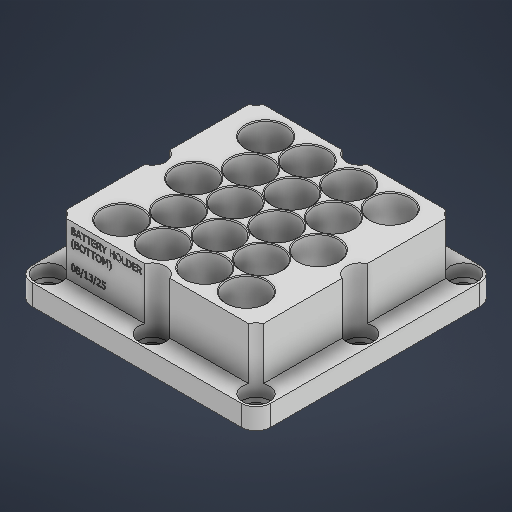
# Autodesk Inventor part: Battery Holder
Saved by Autodesk Inventor 2025 (Build 290162000, 162)
## iProperties
Created: 2025-08-08
Part Number: Battery Holder
Material: Generic
Document SubType Name: Modeling
Designer: mayhe
Density: 1 g/cm^3
Appearance: Default
Author: mayhe
Autodesk Inventor part; units mm, degrees
ref_plane "YZ Plane" through (0, 0, 0) normal (1, 0, 0) x (0, 1, 0)
ref_plane "XZ Plane" through (0, 0, 0) normal (0, 1, 0) x (-1, 0, 0)
ref_plane "XY Plane" through (0, 0, 0) normal (0, 0, 1) x (1, 0, 0)
sketch "Sketch1" plane through (0, 0, 0) normal (0, 1, 0) x (-1, 0, 0)
  line L0 (57.5, 57.5) -> (-57.5, 57.5)
  line L1 (-57.5, 57.5) -> (-57.5, -57.5)
  line L2 (-57.5, -57.5) -> (57.5, -57.5)
  line L3 (57.5, -57.5) -> (57.5, 57.5)
  line L4 (57.5, 57.5) -> (-57.5, -57.5) construction
  line L5 (-57.5, 57.5) -> (57.5, -57.5) construction
  point P0 (0, 0)
  dimension "d0" = 115
  dimension "d1" = 115
  constraints: 12 end point, 2 midpoint, 2 parallel, 1 horizontal, 1 perpendicular
  measures "d0" distance of L2.end L1.end
  measures "d1" distance of L1.end L0.end
extrude "Extrusion1" add sketch "Sketch1" along normal blind 10
sketch "Sketch4" plane through (0, 10, 0) normal (0, 1, 0) x (1, 0, 0)
  line L0 (-47.5, -47.5) -> (47.5, -47.5)
  line L1 (47.5, -47.5) -> (47.5, 47.5)
  line L2 (47.5, 47.5) -> (-47.5, 47.5)
  line L3 (-47.5, 47.5) -> (-47.5, -47.5)
  line L4 (-57.5, 57.5) -> (-57.5, -57.5) projected
  line L5 (-57.5, 0) -> (-47.5, 0)
  line L6 (-30, 34.641) -> (30, 34.641)
  line L7 (30, 34.641) -> (30, -34.641)
  line L8 (30, -34.641) -> (-30, -34.641)
  line L9 (-30, -34.641) -> (-30, 34.641)
  line L10 (-30, 34.641) -> (30, -34.641) construction
  line L11 (30, 34.641) -> (-30, -34.641) construction
  circle A0 centre (-30, 34.641) radius 9.5
  circle A1 centre (-10, 34.641) radius 9.5
  circle A2 centre (10, 34.641) radius 9.5
  circle A3 centre (30, 34.641) radius 9.5
  circle A4 centre (-30, 0) radius 9.5
  circle A5 centre (-10, 0) radius 9.5
  circle A6 centre (10, 0) radius 9.5
  circle A7 centre (30, 0) radius 9.5
  circle A8 centre (-30, -34.641) radius 9.5
  circle A9 centre (-10, -34.641) radius 9.5
  circle A10 centre (10, -34.641) radius 9.5
  circle A11 centre (30, -34.641) radius 9.5
  circle A12 centre (-20, 17.3205) radius 9.5
  circle A13 centre (0, 17.3205) radius 9.5
  circle A14 centre (20, 17.3205) radius 9.5
  circle A15 centre (-20, -17.3205) radius 9.5
  circle A16 centre (0, -17.3205) radius 9.5
  circle A17 centre (20, -17.3205) radius 9.5
  point P0 (47.3285, -94.6135)
  point P1 (-53.5957, 219.1108)
  point P2 (0, 0)
  dimension "d1" = 115
  dimension "d138" = 3
  dimension "d48" = 95
  dimension "d49" = 95
  dimension "d132" = 60
  dimension "d133" = 69.282
  dimension "d134" = 19
  dimension "d137" = 20
  dimension "d140" = 34.641
  dimension "d143" = 19
  dimension "d146" = 10
  dimension "d147" = 17.3205
  dimension "d150" = 20
  dimension "d153" = 34.641
  constraints: 22 end point, 18 centre point, 4 horizontal, 4 midpoint, 4 parallel, 2 perpendicular, 2 vertical, 1 coincident, 32 other
  measures "d48" distance of L2.end L1.end
  measures "d49" distance of L1.end L0.end
  measures "d132" distance of L7.end L8.end
  measures "d133" distance of L6.end L7.end
  measures "d134" diameter of A0
  measures "d137" distance of A0.centre A1.centre
  measures "d140" distance of A0.centre A4.centre
  measures "d143" diameter of A12
  measures "d146" horizontal distance of A1.centre A12.centre
  measures "d147" vertical distance of A12.centre A1.centre
  measures "d150" distance of A12.centre A13.centre
  measures "d153" distance of A12.centre A15.centre
extrude "Extrusion2" add sketch "Sketch4" along normal blind 25 contours L3 L2 L1 L0 | L6 A1 A2 A3 L7 A7 A11 L8 A10 A9 A8 L9 A4 A0
sketch "Sketch5" plane through (0, 35, 0) normal (0, 1, 0) x (1, 0, 0)
  line L0 (50, 50) -> (-50, 50)
  line L1 (-50, 50) -> (-50, -50)
  line L2 (-50, -50) -> (50, -50)
  line L3 (50, -50) -> (50, 50)
  line L4 (50, 50) -> (-50, -50) construction
  line L5 (-50, 50) -> (50, -50) construction
  circle A0 centre (-50, -50) radius 3.5
  circle A1 centre (0, -50) radius 3.5
  circle A2 centre (-50, 0) radius 3.5
  circle A3 centre (0, 0) radius 3.5
  circle A4 centre (50, -50) radius 3.5
  circle A5 centre (50, 0) radius 3.5
  circle A6 centre (-50, 50) radius 3.5
  circle A7 centre (0, 50) radius 3.5
  circle A8 centre (50, 50) radius 3.5
  point P0 (0, 0)
  dimension "d156" = 100
  dimension "d157" = 100
  dimension "d158" = 7
  dimension "d161" = 50
  dimension "d164" = 50
  constraints: 12 end point, 9 centre point, 2 horizontal, 2 midpoint, 2 parallel, 1 coincident, 1 perpendicular, 1 vertical, 16 other
  measures "d156" distance of L2.end L1.end
  measures "d157" distance of L1.end L0.end
  measures "d158" diameter of A0
  measures "d161" distance of A0.centre A1.centre
  measures "d164" distance of A0.centre A2.centre
hole "Hole3" at (-50, 35, 50) at (50, 35, 50) at (-50, 35, -50) at (50, 35, -50) at (-50, 35, 0) at (0, 35, 50) at (50, 35, 0) at (0, 35, -50) direction (0, -1, 0) diameter 7.125 end through all counterbore diameter 13 counterbore depth 31
fillet "Fillet1" radius 7.125 4 edges at (57.5, 5, 57.5) (57.5, 5, -57.5) (-57.5, 5, 57.5) (-57.5, 5, -57.5)
chamfer "Chamfer1" distance 0.4 angle 45 18 edges at (-39.5, 35, -34.641) (-19.5, 35, -34.641) (-29.5, 35, -17.3205) (0.5, 35, -34.641) (20.5, 35, -34.641) (10.5, 35, -17.3205) (-9.5, 35, -17.3205) (-39.5, 35, 0) (-19.5, 35, 0) (0.5, 35, 0) (20.5, 35, 0) (10.5, 35, 17.3205) (-9.5, 35, 17.3205) (-29.5, 35, 17.3205) (-39.5, 35, 34.641) (-19.5, 35, 34.641) (0.5, 35, 34.641) (20.5, 35, 34.641)
sketch "Sketch6" plane through (-44, 10, 47.5) normal (0, 0, 1) x (1, 0, 0)
  line L0 (2.3115, 22.6775) -> (39.9401, 22.6775) construction
  line L1 (39.9401, 22.6775) -> (39.9401, -1.6821) construction
  line L2 (39.9401, -1.6821) -> (2.3115, -1.6821) construction
  line L3 (2.3115, -1.6821) -> (2.3115, 22.6775) construction
  spline S0 degree 2 poles (4.6876, 20.5014) (4.6876, 20.2741) (4.5147, 19.9259) (4.3715, 19.8123) knots 0 0 0 1 2 2 2
  spline S1 degree 2 poles (4.3715, 19.8123) (4.1986, 19.6789) (3.8058, 19.5653) (3.4946, 19.5653) knots 0 0 0 1 2 2 2
  line L4 (3.4946, 19.5653) -> (2.6202, 19.5653)
  line L5 (2.6202, 19.5653) -> (2.6202, 22.6133)
  line L6 (2.6202, 22.6133) -> (3.4279, 22.6133)
  spline S2 degree 2 poles (3.4279, 22.6133) (3.754, 22.6133) (4.08, 22.5713) (4.2282, 22.4898) knots 0 0 0 1 2 2 2
  spline S3 degree 2 poles (4.2282, 22.4898) (4.3937, 22.4033) (4.5444, 22.1193) (4.5444, 21.9266) knots 0 0 0 1 2 2 2
  spline S4 degree 2 poles (4.5444, 21.9266) (4.5444, 21.7117) (4.3171, 21.3708) (4.117, 21.2745) knots 0 0 0 1 2 2 2
  line L7 (4.117, 21.2745) -> (4.117, 21.2597)
  spline S5 degree 2 poles (4.117, 21.2597) (4.3887, 21.1856) (4.6876, 20.7929) (4.6876, 20.5014) knots 0 0 0 1 2 2 2
  spline S6 degree 2 poles (4.2652, 20.4841) (4.2652, 20.657) (4.1664, 20.8793) (4.0182, 20.9583) knots 0 0 0 1 2 2 2
  spline S7 degree 2 poles (4.0182, 20.9583) (3.9219, 21.0077) (3.6947, 21.0374) (3.4847, 21.0374) knots 0 0 0 1 2 2 2
  line L8 (3.4847, 21.0374) -> (3.0253, 21.0374)
  line L9 (3.0253, 21.0374) -> (3.0253, 19.9111)
  line L10 (3.0253, 19.9111) -> (3.3538, 19.9111)
  spline S8 degree 2 poles (3.3538, 19.9111) (3.6206, 19.9111) (3.9269, 19.9605) (4.0454, 20.0395) knots 0 0 0 1 2 2 2
  spline S9 degree 2 poles (4.0454, 20.0395) (4.159, 20.121) (4.2652, 20.3235) (4.2652, 20.4841) knots 0 0 0 1 2 2 2
  spline S10 degree 2 poles (4.122, 21.8698) (4.122, 21.9785) (4.0479, 22.1415) (3.9664, 22.1884) knots 0 0 0 1 2 2 2
  spline S11 degree 2 poles (3.9664, 22.1884) (3.8676, 22.2428) (3.628, 22.2675) (3.4131, 22.2675) knots 0 0 0 1 2 2 2
  line L11 (3.4131, 22.2675) -> (3.0253, 22.2675)
  line L12 (3.0253, 22.2675) -> (3.0253, 21.3758)
  line L13 (3.0253, 21.3758) -> (3.4847, 21.3758)
  spline S12 degree 2 poles (3.4847, 21.3758) (3.6749, 21.3758) (3.8552, 21.4153) (3.9516, 21.477) knots 0 0 0 1 2 2 2
  spline S13 degree 2 poles (3.9516, 21.477) (4.0454, 21.5363) (4.122, 21.7265) (4.122, 21.8698) knots 0 0 0 1 2 2 2
  line L14 (4.7617, 19.5653) -> (5.7892, 22.6133)
  line L15 (5.7892, 22.6133) -> (6.2882, 22.6133)
  line L16 (6.2882, 22.6133) -> (7.3157, 19.5653)
  line L17 (7.3157, 19.5653) -> (6.8884, 19.5653)
  line L18 (6.8884, 19.5653) -> (6.6118, 20.4174)
  line L19 (6.6118, 20.4174) -> (5.4484, 20.4174)
  line L20 (5.4484, 20.4174) -> (5.1717, 19.5653)
  line L21 (5.1717, 19.5653) -> (4.7617, 19.5653)
  line L22 (6.5006, 20.7632) -> (6.0288, 22.1983)
  line L23 (6.0288, 22.1983) -> (5.5595, 20.7632)
  line L24 (5.5595, 20.7632) -> (6.5006, 20.7632)
  line L25 (8.3161, 19.5653) -> (8.3161, 22.2526)
  line L26 (8.3161, 22.2526) -> (7.2935, 22.2526)
  line L27 (7.2935, 22.2526) -> (7.2935, 22.6133)
  line L28 (7.2935, 22.6133) -> (9.7437, 22.6133)
  line L29 (9.7437, 22.6133) -> (9.7437, 22.2526)
  line L30 (9.7437, 22.2526) -> (8.7212, 22.2526)
  line L31 (8.7212, 22.2526) -> (8.7212, 19.5653)
  line L32 (8.7212, 19.5653) -> (8.3161, 19.5653)
  line L33 (10.7639, 19.5653) -> (10.7639, 22.2526)
  line L34 (10.7639, 22.2526) -> (9.7413, 22.2526)
  line L35 (9.7413, 22.2526) -> (9.7413, 22.6133)
  line L36 (9.7413, 22.6133) -> (12.1915, 22.6133)
  line L37 (12.1915, 22.6133) -> (12.1915, 22.2526)
  line L38 (12.1915, 22.2526) -> (11.1689, 22.2526)
  line L39 (11.1689, 22.2526) -> (11.1689, 19.5653)
  line L40 (11.1689, 19.5653) -> (10.7639, 19.5653)
  line L41 (12.5003, 19.5653) -> (12.5003, 22.6133)
  line L42 (12.5003, 22.6133) -> (14.4071, 22.6133)
  line L43 (14.4071, 22.6133) -> (14.4071, 22.2526)
  line L44 (14.4071, 22.2526) -> (12.9054, 22.2526)
  line L45 (12.9054, 22.2526) -> (12.9054, 21.4178)
  line L46 (12.9054, 21.4178) -> (14.3059, 21.4178)
  line L47 (14.3059, 21.4178) -> (14.3059, 21.0571)
  line L48 (14.3059, 21.0571) -> (12.9054, 21.0571)
  line L49 (12.9054, 21.0571) -> (12.9054, 19.9259)
  line L50 (12.9054, 19.9259) -> (14.4071, 19.9259)
  line L51 (14.4071, 19.9259) -> (14.4071, 19.5653)
  line L52 (14.4071, 19.5653) -> (12.5003, 19.5653)
  line L53 (17.2106, 19.5653) -> (16.6845, 19.5653)
  line L54 (16.6845, 19.5653) -> (15.7212, 20.778)
  line L55 (15.7212, 20.778) -> (15.2568, 20.778)
  line L56 (15.2568, 20.778) -> (15.2568, 19.5653)
  line L57 (15.2568, 19.5653) -> (14.8517, 19.5653)
  line L58 (14.8517, 19.5653) -> (14.8517, 22.6133)
  line L59 (14.8517, 22.6133) -> (15.6372, 22.6133)
  spline S14 degree 2 poles (15.6372, 22.6133) (15.899, 22.6133) (16.2522, 22.5564) (16.4128, 22.4527) knots 0 0 0 1 2 2 2
  spline S15 degree 2 poles (16.4128, 22.4527) (16.5733, 22.349) (16.7586, 22.0254) (16.7586, 21.7858) knots 0 0 0 1 2 2 2
  spline S16 degree 2 poles (16.7586, 21.7858) (16.7586, 21.4523) (16.4177, 21.0003) (16.1263, 20.8917) knots 0 0 0 1 2 2 2
  line L60 (16.1263, 20.8917) -> (17.2106, 19.5653)
  spline S17 degree 2 poles (16.3362, 21.7537) (16.3362, 21.8871) (16.2424, 22.0921) (16.1436, 22.1588) knots 0 0 0 1 2 2 2
  spline S18 degree 2 poles (16.1436, 22.1588) (16.0571, 22.2156) (15.8274, 22.2625) (15.6594, 22.2625) knots 0 0 0 1 2 2 2
  line L61 (15.6594, 22.2625) -> (15.2568, 22.2625)
  line L62 (15.2568, 22.2625) -> (15.2568, 21.1164)
  line L63 (15.2568, 21.1164) -> (15.6125, 21.1164)
  spline S19 degree 2 poles (15.6125, 21.1164) (15.7879, 21.1164) (16.067, 21.1782) (16.1633, 21.2745) knots 0 0 0 1 2 2 2
  spline S20 degree 2 poles (16.1633, 21.2745) (16.2522, 21.3585) (16.3362, 21.5956) (16.3362, 21.7537) knots 0 0 0 1 2 2 2
  line L64 (19.5868, 22.6133) -> (18.5568, 20.9139)
  line L65 (18.5568, 20.9139) -> (18.5568, 19.5653)
  line L66 (18.5568, 19.5653) -> (18.1517, 19.5653)
  line L67 (18.1517, 19.5653) -> (18.1517, 20.8719)
  line L68 (18.1517, 20.8719) -> (17.1217, 22.6133)
  line L69 (17.1217, 22.6133) -> (17.5712, 22.6133)
  line L70 (17.5712, 22.6133) -> (18.3592, 21.272)
  line L71 (18.3592, 21.272) -> (19.157, 22.6133)
  line L72 (19.157, 22.6133) -> (19.5868, 22.6133)
  line L73 (23.3906, 19.5653) -> (22.9855, 19.5653)
  line L74 (22.9855, 19.5653) -> (22.9855, 21.0571)
  line L75 (22.9855, 21.0571) -> (21.5825, 21.0571)
  line L76 (21.5825, 21.0571) -> (21.5825, 19.5653)
  line L77 (21.5825, 19.5653) -> (21.1774, 19.5653)
  line L78 (21.1774, 19.5653) -> (21.1774, 22.6133)
  line L79 (21.1774, 22.6133) -> (21.5825, 22.6133)
  line L80 (21.5825, 22.6133) -> (21.5825, 21.4178)
  line L81 (21.5825, 21.4178) -> (22.9855, 21.4178)
  line L82 (22.9855, 21.4178) -> (22.9855, 22.6133)
  line L83 (22.9855, 22.6133) -> (23.3906, 22.6133)
  line L84 (23.3906, 22.6133) -> (23.3906, 19.5653)
  spline S21 degree 2 poles (26.1644, 22.265) (26.3373, 22.0624) (26.53, 21.4696) (26.53, 21.0893) knots 0 0 0 1 2 2 2
  spline S22 degree 2 poles (26.53, 21.0893) (26.53, 20.7188) (26.3423, 20.1185) (26.1644, 19.916) knots 0 0 0 1 2 2 2
  spline S23 degree 2 poles (26.1644, 19.916) (25.9767, 19.7036) (25.4802, 19.501) (25.1813, 19.501) knots 0 0 0 1 2 2 2
  spline S24 degree 2 poles (25.1813, 19.501) (24.8726, 19.501) (24.3786, 19.711) (24.1983, 19.916) knots 0 0 0 1 2 2 2
  spline S25 degree 2 poles (24.1983, 19.916) (24.0229, 20.1185) (23.8352, 20.7138) (23.8352, 21.0893) knots 0 0 0 1 2 2 2
  spline S26 degree 2 poles (23.8352, 21.0893) (23.8352, 21.4721) (24.0254, 22.055) (24.2007, 22.265) knots 0 0 0 1 2 2 2
  spline S27 degree 2 poles (24.2007, 22.265) (24.3786, 22.4675) (24.8751, 22.6775) (25.1813, 22.6775) knots 0 0 0 1 2 2 2
  spline S28 degree 2 poles (25.1813, 22.6775) (25.4926, 22.6775) (25.9915, 22.4601) (26.1644, 22.265) knots 0 0 0 1 2 2 2
  spline S29 degree 2 poles (26.1076, 21.0893) (26.1076, 21.3906) (25.9767, 21.8574) (25.8581, 22.0106) knots 0 0 0 1 2 2 2
  spline S30 degree 2 poles (25.8581, 22.0106) (25.7371, 22.1687) (25.3962, 22.3267) (25.1838, 22.3267) knots 0 0 0 1 2 2 2
  spline S31 degree 2 poles (25.1838, 22.3267) (24.964, 22.3267) (24.633, 22.1736) (24.507, 22.0106) knots 0 0 0 1 2 2 2
  spline S32 degree 2 poles (24.507, 22.0106) (24.386, 21.855) (24.2576, 21.3857) (24.2576, 21.0893) knots 0 0 0 1 2 2 2
  spline S33 degree 2 poles (24.2576, 21.0893) (24.2576, 20.489) (24.7614, 19.8518) (25.1838, 19.8518) knots 0 0 0 1 2 2 2
  spline S34 degree 2 poles (25.1838, 19.8518) (25.6062, 19.8518) (26.1076, 20.489) (26.1076, 21.0893) knots 0 0 0 1 2 2 2
  line L85 (28.7406, 19.5653) -> (26.9746, 19.5653)
  line L86 (26.9746, 19.5653) -> (26.9746, 22.6133)
  line L87 (26.9746, 22.6133) -> (27.3797, 22.6133)
  line L88 (27.3797, 22.6133) -> (27.3797, 19.9259)
  line L89 (27.3797, 19.9259) -> (28.7406, 19.9259)
  line L90 (28.7406, 19.9259) -> (28.7406, 19.5653)
  spline S35 degree 2 poles (31.4626, 21.0868) (31.4626, 20.6694) (31.1242, 19.9975) (30.8402, 19.8098) knots 0 0 0 1 2 2 2
  spline S36 degree 2 poles (30.8402, 19.8098) (30.608, 19.6641) (30.1313, 19.5653) (29.7608, 19.5653) knots 0 0 0 1 2 2 2
  line L91 (29.7608, 19.5653) -> (29.0593, 19.5653)
  line L92 (29.0593, 19.5653) -> (29.0593, 22.6133)
  line L93 (29.0593, 22.6133) -> (29.7533, 22.6133)
  spline S37 degree 2 poles (29.7533, 22.6133) (30.1831, 22.6133) (30.6722, 22.4848) (30.8451, 22.3712) knots 0 0 0 1 2 2 2
  spline S38 degree 2 poles (30.8451, 22.3712) (31.139, 22.1761) (31.4626, 21.5314) (31.4626, 21.0868) knots 0 0 0 1 2 2 2
  spline S39 degree 2 poles (31.0402, 21.0917) (31.0402, 21.4425) (30.808, 21.9389) (30.5783, 22.0797) knots 0 0 0 1 2 2 2
  spline S40 degree 2 poles (30.5783, 22.0797) (30.4153, 22.1761) (30.0473, 22.2625) (29.7731, 22.2625) knots 0 0 0 1 2 2 2
  line L94 (29.7731, 22.2625) -> (29.4644, 22.2625)
  line L95 (29.4644, 22.2625) -> (29.4644, 19.916)
  line L96 (29.4644, 19.916) -> (29.7731, 19.916)
  spline S41 degree 2 poles (29.7731, 19.916) (30.0423, 19.916) (30.4499, 20.0024) (30.6154, 20.1185) knots 0 0 0 1 2 2 2
  spline S42 degree 2 poles (30.6154, 20.1185) (30.8278, 20.2618) (31.0402, 20.736) (31.0402, 21.0917) knots 0 0 0 1 2 2 2
  line L97 (31.9023, 19.5653) -> (31.9023, 22.6133)
  line L98 (31.9023, 22.6133) -> (33.8091, 22.6133)
  line L99 (33.8091, 22.6133) -> (33.8091, 22.2526)
  line L100 (33.8091, 22.2526) -> (32.3073, 22.2526)
  line L101 (32.3073, 22.2526) -> (32.3073, 21.4178)
  line L102 (32.3073, 21.4178) -> (33.7078, 21.4178)
  line L103 (33.7078, 21.4178) -> (33.7078, 21.0571)
  line L104 (33.7078, 21.0571) -> (32.3073, 21.0571)
  line L105 (32.3073, 21.0571) -> (32.3073, 19.9259)
  line L106 (32.3073, 19.9259) -> (33.8091, 19.9259)
  line L107 (33.8091, 19.9259) -> (33.8091, 19.5653)
  line L108 (33.8091, 19.5653) -> (31.9023, 19.5653)
  line L109 (36.6126, 19.5653) -> (36.0865, 19.5653)
  line L110 (36.0865, 19.5653) -> (35.1232, 20.778)
  line L111 (35.1232, 20.778) -> (34.6588, 20.778)
  line L112 (34.6588, 20.778) -> (34.6588, 19.5653)
  line L113 (34.6588, 19.5653) -> (34.2537, 19.5653)
  line L114 (34.2537, 19.5653) -> (34.2537, 22.6133)
  line L115 (34.2537, 22.6133) -> (35.0392, 22.6133)
  spline S43 degree 2 poles (35.0392, 22.6133) (35.301, 22.6133) (35.6542, 22.5564) (35.8148, 22.4527) knots 0 0 0 1 2 2 2
  spline S44 degree 2 poles (35.8148, 22.4527) (35.9753, 22.349) (36.1606, 22.0254) (36.1606, 21.7858) knots 0 0 0 1 2 2 2
  spline S45 degree 2 poles (36.1606, 21.7858) (36.1606, 21.4523) (35.8197, 21.0003) (35.5282, 20.8917) knots 0 0 0 1 2 2 2
  line L116 (35.5282, 20.8917) -> (36.6126, 19.5653)
  spline S46 degree 2 poles (35.7382, 21.7537) (35.7382, 21.8871) (35.6443, 22.0921) (35.5455, 22.1588) knots 0 0 0 1 2 2 2
  spline S47 degree 2 poles (35.5455, 22.1588) (35.4591, 22.2156) (35.2294, 22.2625) (35.0614, 22.2625) knots 0 0 0 1 2 2 2
  line L117 (35.0614, 22.2625) -> (34.6588, 22.2625)
  line L118 (34.6588, 22.2625) -> (34.6588, 21.1164)
  line L119 (34.6588, 21.1164) -> (35.0145, 21.1164)
  spline S48 degree 2 poles (35.0145, 21.1164) (35.1899, 21.1164) (35.469, 21.1782) (35.5653, 21.2745) knots 0 0 0 1 2 2 2
  spline S49 degree 2 poles (35.5653, 21.2745) (35.6542, 21.3585) (35.7382, 21.5956) (35.7382, 21.7537) knots 0 0 0 1 2 2 2
  line L120 (3.7638, 13.7045) -> (3.2945, 13.7045)
  spline S50 degree 2 poles (3.2945, 13.7045) (2.9389, 14.1269) (2.5313, 15.0729) (2.5313, 15.7176) knots 0 0 0 1 2 2 2
  spline S51 degree 2 poles (2.5313, 15.7176) (2.5313, 16.3474) (2.9339, 17.3083) (3.2945, 17.7307) knots 0 0 0 1 2 2 2
  line L121 (3.2945, 17.7307) -> (3.7638, 17.7307)
  line L122 (3.7638, 17.7307) -> (3.7638, 17.7109)
  spline S52 degree 2 poles (3.7638, 17.7109) (3.5983, 17.5602) (3.297, 17.17) (3.1686, 16.9106) knots 0 0 0 1 2 2 2
  spline S53 degree 2 poles (3.1686, 16.9106) (3.0451, 16.6587) (2.8919, 16.0535) (2.8919, 15.7176) knots 0 0 0 1 2 2 2
  spline S54 degree 2 poles (2.8919, 15.7176) (2.8919, 15.3668) (3.0401, 14.7864) (3.1686, 14.5246) knots 0 0 0 1 2 2 2
  spline S55 degree 2 poles (3.1686, 14.5246) (3.2921, 14.2726) (3.6058, 13.8651) (3.7638, 13.7243) knots 0 0 0 1 2 2 2
  line L123 (3.7638, 13.7243) -> (3.7638, 13.7045)
  spline S56 degree 2 poles (6.2931, 15.4829) (6.2931, 15.2557) (6.1202, 14.9074) (5.977, 14.7938) knots 0 0 0 1 2 2 2
  spline S57 degree 2 poles (5.977, 14.7938) (5.8041, 14.6604) (5.4113, 14.5468) (5.1001, 14.5468) knots 0 0 0 1 2 2 2
  line L124 (5.1001, 14.5468) -> (4.2257, 14.5468)
  line L125 (4.2257, 14.5468) -> (4.2257, 17.5948)
  line L126 (4.2257, 17.5948) -> (5.0334, 17.5948)
  spline S58 degree 2 poles (5.0334, 17.5948) (5.3595, 17.5948) (5.6855, 17.5528) (5.8337, 17.4713) knots 0 0 0 1 2 2 2
  spline S59 degree 2 poles (5.8337, 17.4713) (5.9992, 17.3849) (6.1499, 17.1008) (6.1499, 16.9081) knots 0 0 0 1 2 2 2
  spline S60 degree 2 poles (6.1499, 16.9081) (6.1499, 16.6932) (5.9226, 16.3524) (5.7226, 16.2561) knots 0 0 0 1 2 2 2
  line L127 (5.7226, 16.2561) -> (5.7226, 16.2412)
  spline S61 degree 2 poles (5.7226, 16.2412) (5.9943, 16.1671) (6.2931, 15.7744) (6.2931, 15.4829) knots 0 0 0 1 2 2 2
  spline S62 degree 2 poles (5.8708, 15.4656) (5.8708, 15.6385) (5.772, 15.8609) (5.6238, 15.9399) knots 0 0 0 1 2 2 2
  spline S63 degree 2 poles (5.6238, 15.9399) (5.5274, 15.9893) (5.3002, 16.0189) (5.0902, 16.0189) knots 0 0 0 1 2 2 2
  line L128 (5.0902, 16.0189) -> (4.6308, 16.0189)
  line L129 (4.6308, 16.0189) -> (4.6308, 14.8926)
  line L130 (4.6308, 14.8926) -> (4.9593, 14.8926)
  spline S64 degree 2 poles (4.9593, 14.8926) (5.2261, 14.8926) (5.5324, 14.942) (5.6509, 15.021) knots 0 0 0 1 2 2 2
  spline S65 degree 2 poles (5.6509, 15.021) (5.7645, 15.1026) (5.8708, 15.3051) (5.8708, 15.4656) knots 0 0 0 1 2 2 2
  spline S66 degree 2 poles (5.7275, 16.8513) (5.7275, 16.96) (5.6534, 17.123) (5.5719, 17.17) knots 0 0 0 1 2 2 2
  spline S67 degree 2 poles (5.5719, 17.17) (5.4731, 17.2243) (5.2335, 17.249) (5.0186, 17.249) knots 0 0 0 1 2 2 2
  line L131 (5.0186, 17.249) -> (4.6308, 17.249)
  line L132 (4.6308, 17.249) -> (4.6308, 16.3573)
  line L133 (4.6308, 16.3573) -> (5.0902, 16.3573)
  spline S68 degree 2 poles (5.0902, 16.3573) (5.2804, 16.3573) (5.4607, 16.3968) (5.5571, 16.4586) knots 0 0 0 1 2 2 2
  spline S69 degree 2 poles (5.5571, 16.4586) (5.6509, 16.5179) (5.7275, 16.7081) (5.7275, 16.8513) knots 0 0 0 1 2 2 2
  spline S70 degree 2 poles (8.8521, 17.2465) (9.025, 17.044) (9.2176, 16.4512) (9.2176, 16.0708) knots 0 0 0 1 2 2 2
  spline S71 degree 2 poles (9.2176, 16.0708) (9.2176, 15.7003) (9.0299, 15.1001) (8.8521, 14.8975) knots 0 0 0 1 2 2 2
  spline S72 degree 2 poles (8.8521, 14.8975) (8.6643, 14.6851) (8.1679, 14.4826) (7.869, 14.4826) knots 0 0 0 1 2 2 2
  spline S73 degree 2 poles (7.869, 14.4826) (7.5603, 14.4826) (7.0662, 14.6925) (6.8859, 14.8975) knots 0 0 0 1 2 2 2
  spline S74 degree 2 poles (6.8859, 14.8975) (6.7106, 15.1001) (6.5228, 15.6954) (6.5228, 16.0708) knots 0 0 0 1 2 2 2
  spline S75 degree 2 poles (6.5228, 16.0708) (6.5228, 16.4537) (6.713, 17.0366) (6.8884, 17.2465) knots 0 0 0 1 2 2 2
  spline S76 degree 2 poles (6.8884, 17.2465) (7.0662, 17.4491) (7.5627, 17.659) (7.869, 17.659) knots 0 0 0 1 2 2 2
  spline S77 degree 2 poles (7.869, 17.659) (8.1802, 17.659) (8.6792, 17.4417) (8.8521, 17.2465) knots 0 0 0 1 2 2 2
  spline S78 degree 2 poles (8.7953, 16.0708) (8.7953, 16.3721) (8.6643, 16.839) (8.5458, 16.9921) knots 0 0 0 1 2 2 2
  spline S79 degree 2 poles (8.5458, 16.9921) (8.4248, 17.1502) (8.0839, 17.3083) (7.8715, 17.3083) knots 0 0 0 1 2 2 2
  spline S80 degree 2 poles (7.8715, 17.3083) (7.6516, 17.3083) (7.3207, 17.1551) (7.1947, 16.9921) knots 0 0 0 1 2 2 2
  spline S81 degree 2 poles (7.1947, 16.9921) (7.0737, 16.8365) (6.9452, 16.3672) (6.9452, 16.0708) knots 0 0 0 1 2 2 2
  spline S82 degree 2 poles (6.9452, 16.0708) (6.9452, 15.4706) (7.4491, 14.8333) (7.8715, 14.8333) knots 0 0 0 1 2 2 2
  spline S83 degree 2 poles (7.8715, 14.8333) (8.2938, 14.8333) (8.7953, 15.4706) (8.7953, 16.0708) knots 0 0 0 1 2 2 2
  line L134 (10.3736, 14.5468) -> (10.3736, 17.2342)
  line L135 (10.3736, 17.2342) -> (9.351, 17.2342)
  line L136 (9.351, 17.2342) -> (9.351, 17.5948)
  line L137 (9.351, 17.5948) -> (11.8013, 17.5948)
  line L138 (11.8013, 17.5948) -> (11.8013, 17.2342)
  line L139 (11.8013, 17.2342) -> (10.7787, 17.2342)
  line L140 (10.7787, 17.2342) -> (10.7787, 14.5468)
  line L141 (10.7787, 14.5468) -> (10.3736, 14.5468)
  line L142 (12.8214, 14.5468) -> (12.8214, 17.2342)
  line L143 (12.8214, 17.2342) -> (11.7988, 17.2342)
  line L144 (11.7988, 17.2342) -> (11.7988, 17.5948)
  line L145 (11.7988, 17.5948) -> (14.2491, 17.5948)
  line L146 (14.2491, 17.5948) -> (14.2491, 17.2342)
  line L147 (14.2491, 17.2342) -> (13.2265, 17.2342)
  line L148 (13.2265, 17.2342) -> (13.2265, 14.5468)
  line L149 (13.2265, 14.5468) -> (12.8214, 14.5468)
  spline S84 degree 2 poles (16.7141, 17.2465) (16.887, 17.044) (17.0797, 16.4512) (17.0797, 16.0708) knots 0 0 0 1 2 2 2
  spline S85 degree 2 poles (17.0797, 16.0708) (17.0797, 15.7003) (16.892, 15.1001) (16.7141, 14.8975) knots 0 0 0 1 2 2 2
  spline S86 degree 2 poles (16.7141, 14.8975) (16.5264, 14.6851) (16.0299, 14.4826) (15.7311, 14.4826) knots 0 0 0 1 2 2 2
  spline S87 degree 2 poles (15.7311, 14.4826) (15.4223, 14.4826) (14.9283, 14.6925) (14.748, 14.8975) knots 0 0 0 1 2 2 2
  spline S88 degree 2 poles (14.748, 14.8975) (14.5726, 15.1001) (14.3849, 15.6954) (14.3849, 16.0708) knots 0 0 0 1 2 2 2
  spline S89 degree 2 poles (14.3849, 16.0708) (14.3849, 16.4537) (14.5751, 17.0366) (14.7505, 17.2465) knots 0 0 0 1 2 2 2
  spline S90 degree 2 poles (14.7505, 17.2465) (14.9283, 17.4491) (15.4248, 17.659) (15.7311, 17.659) knots 0 0 0 1 2 2 2
  spline S91 degree 2 poles (15.7311, 17.659) (16.0423, 17.659) (16.5412, 17.4417) (16.7141, 17.2465) knots 0 0 0 1 2 2 2
  spline S92 degree 2 poles (16.6573, 16.0708) (16.6573, 16.3721) (16.5264, 16.839) (16.4078, 16.9921) knots 0 0 0 1 2 2 2
  spline S93 degree 2 poles (16.4078, 16.9921) (16.2868, 17.1502) (15.946, 17.3083) (15.7335, 17.3083) knots 0 0 0 1 2 2 2
  spline S94 degree 2 poles (15.7335, 17.3083) (15.5137, 17.3083) (15.1827, 17.1551) (15.0567, 16.9921) knots 0 0 0 1 2 2 2
  spline S95 degree 2 poles (15.0567, 16.9921) (14.9357, 16.8365) (14.8073, 16.3672) (14.8073, 16.0708) knots 0 0 0 1 2 2 2
  spline S96 degree 2 poles (14.8073, 16.0708) (14.8073, 15.4706) (15.3112, 14.8333) (15.7335, 14.8333) knots 0 0 0 1 2 2 2
  spline S97 degree 2 poles (15.7335, 14.8333) (16.1559, 14.8333) (16.6573, 15.4706) (16.6573, 16.0708) knots 0 0 0 1 2 2 2
  line L150 (20.1376, 14.5468) -> (19.7325, 14.5468)
  line L151 (19.7325, 14.5468) -> (19.7325, 17.1724)
  line L152 (19.7325, 17.1724) -> (18.9371, 15.3866)
  line L153 (18.9371, 15.3866) -> (18.6901, 15.3866)
  line L154 (18.6901, 15.3866) -> (17.9022, 17.1724)
  line L155 (17.9022, 17.1724) -> (17.9022, 14.5468)
  line L156 (17.9022, 14.5468) -> (17.5243, 14.5468)
  line L157 (17.5243, 14.5468) -> (17.5243, 17.5948)
  line L158 (17.5243, 17.5948) -> (18.0776, 17.5948)
  line L159 (18.0776, 17.5948) -> (18.8383, 15.8979)
  line L160 (18.8383, 15.8979) -> (19.5744, 17.5948)
  line L161 (19.5744, 17.5948) -> (20.1376, 17.5948)
  line L162 (20.1376, 17.5948) -> (20.1376, 14.5468)
  spline S98 degree 2 poles (21.832, 15.7176) (21.832, 15.0853) (21.4269, 14.1269) (21.0688, 13.7045) knots 0 0 0 1 2 2 2
  line L163 (21.0688, 13.7045) -> (20.5995, 13.7045)
  line L164 (20.5995, 13.7045) -> (20.5995, 13.7243)
  spline S99 degree 2 poles (20.5995, 13.7243) (20.7575, 13.8651) (21.0762, 14.2776) (21.1947, 14.5246) knots 0 0 0 1 2 2 2
  spline S100 degree 2 poles (21.1947, 14.5246) (21.3232, 14.7889) (21.4714, 15.3767) (21.4714, 15.7176) knots 0 0 0 1 2 2 2
  spline S101 degree 2 poles (21.4714, 15.7176) (21.4714, 16.056) (21.3207, 16.6562) (21.1947, 16.9106) knots 0 0 0 1 2 2 2
  spline S102 degree 2 poles (21.1947, 16.9106) (21.0712, 17.165) (20.7551, 17.5701) (20.5995, 17.7109) knots 0 0 0 1 2 2 2
  line L165 (20.5995, 17.7109) -> (20.5995, 17.7307)
  line L166 (20.5995, 17.7307) -> (21.0688, 17.7307)
  spline S103 degree 2 poles (21.0688, 17.7307) (21.4245, 17.3083) (21.832, 16.3549) (21.832, 15.7176) knots 0 0 0 1 2 2 2
  spline S104 degree 2 poles (4.4307, 6.0339) (4.4307, 5.2139) (3.954, 4.4457) (3.4576, 4.4457) knots 0 0 0 1 2 2 2
  spline S105 degree 2 poles (3.4576, 4.4457) (2.9537, 4.4457) (2.4819, 5.2287) (2.4819, 6.0314) knots 0 0 0 1 2 2 2
  spline S106 degree 2 poles (2.4819, 6.0314) (2.4819, 6.8564) (2.9586, 7.6196) (3.4576, 7.6196) knots 0 0 0 1 2 2 2
  spline S107 degree 2 poles (3.4576, 7.6196) (3.959, 7.6196) (4.4307, 6.8292) (4.4307, 6.0339) knots 0 0 0 1 2 2 2
  spline S108 degree 2 poles (3.9071, 5.1052) (3.9664, 5.2558) (4.0158, 5.7202) (4.0158, 6.0339) knots 0 0 0 1 2 2 2
  spline S109 degree 2 poles (4.0158, 6.0339) (4.0158, 6.3476) (3.9664, 6.8095) (3.9046, 6.9651) knots 0 0 0 1 2 2 2
  spline S110 degree 2 poles (3.9046, 6.9651) (3.8429, 7.1207) (3.628, 7.2813) (3.4576, 7.2813) knots 0 0 0 1 2 2 2
  spline S111 degree 2 poles (3.4576, 7.2813) (3.2871, 7.2813) (3.0673, 7.1207) (3.0031, 6.9602) knots 0 0 0 1 2 2 2
  spline S112 degree 2 poles (3.0031, 6.9602) (2.9413, 6.8045) (2.8969, 6.3303) (2.8969, 6.0314) knots 0 0 0 1 2 2 2
  spline S113 degree 2 poles (2.8969, 6.0314) (2.8969, 5.7103) (2.9364, 5.2805) (3.0006, 5.1126) knots 0 0 0 1 2 2 2
  spline S114 degree 2 poles (3.0006, 5.1126) (3.0599, 4.9545) (3.2797, 4.7841) (3.4576, 4.7841) knots 0 0 0 1 2 2 2
  spline S115 degree 2 poles (3.4576, 4.7841) (3.6255, 4.7841) (3.8453, 4.9446) (3.9071, 5.1052) knots 0 0 0 1 2 2 2
  spline S116 degree 2 poles (5.7423, 4.4407) (5.5151, 4.4407) (5.1421, 4.5766) (5.0112, 4.7026) knots 0 0 0 1 2 2 2
  spline S117 degree 2 poles (5.0112, 4.7026) (4.8828, 4.8261) (4.7494, 5.162) (4.7494, 5.3522) knots 0 0 0 1 2 2 2
  spline S118 degree 2 poles (4.7494, 5.3522) (4.7494, 5.5992) (5.0137, 6.0141) (5.2656, 6.1376) knots 0 0 0 1 2 2 2
  line L167 (5.2656, 6.1376) -> (5.2656, 6.15)
  spline S119 degree 2 poles (5.2656, 6.15) (5.0408, 6.2809) (4.8235, 6.5921) (4.8235, 6.8243) knots 0 0 0 1 2 2 2
  spline S120 degree 2 poles (4.8235, 6.8243) (4.8235, 7.1676) (5.3422, 7.6271) (5.7423, 7.6271) knots 0 0 0 1 2 2 2
  spline S121 degree 2 poles (5.7423, 7.6271) (6.1573, 7.6271) (6.6587, 7.1923) (6.6587, 6.8515) knots 0 0 0 1 2 2 2
  spline S122 degree 2 poles (6.6587, 6.8515) (6.6587, 6.6465) (6.4191, 6.2463) (6.1943, 6.1327) knots 0 0 0 1 2 2 2
  line L168 (6.1943, 6.1327) -> (6.1943, 6.1203)
  spline S123 degree 2 poles (6.1943, 6.1203) (6.4611, 5.9968) (6.7353, 5.6412) (6.7353, 5.3596) knots 0 0 0 1 2 2 2
  spline S124 degree 2 poles (6.7353, 5.3596) (6.7353, 4.9693) (6.1672, 4.4407) (5.7423, 4.4407) knots 0 0 0 1 2 2 2
  spline S125 degree 2 poles (6.3154, 5.3201) (6.3154, 5.5078) (6.1672, 5.7301) (5.9572, 5.8437) knots 0 0 0 1 2 2 2
  spline S126 degree 2 poles (5.9572, 5.8437) (5.888, 5.8832) (5.6559, 5.9746) (5.5101, 6.0339) knots 0 0 0 1 2 2 2
  spline S127 degree 2 poles (5.5101, 6.0339) (5.3422, 5.9227) (5.1619, 5.5918) (5.1619, 5.3818) knots 0 0 0 1 2 2 2
  spline S128 degree 2 poles (5.1619, 5.3818) (5.1619, 5.1052) (5.4953, 4.7446) (5.7473, 4.7446) knots 0 0 0 1 2 2 2
  spline S129 degree 2 poles (5.7473, 4.7446) (6.0041, 4.7446) (6.3154, 5.0533) (6.3154, 5.3201) knots 0 0 0 1 2 2 2
  spline S130 degree 2 poles (6.2586, 6.8465) (6.2586, 7.0515) (5.9844, 7.3257) (5.7398, 7.3257) knots 0 0 0 1 2 2 2
  spline S131 degree 2 poles (5.7398, 7.3257) (5.5175, 7.3257) (5.2335, 7.0812) (5.2335, 6.8712) knots 0 0 0 1 2 2 2
  spline S132 degree 2 poles (5.2335, 6.8712) (5.2335, 6.7206) (5.3792, 6.5106) (5.525, 6.4266) knots 0 0 0 1 2 2 2
  spline S133 degree 2 poles (5.525, 6.4266) (5.5867, 6.3921) (5.8485, 6.271) (5.9547, 6.2364) knots 0 0 0 1 2 2 2
  spline S134 degree 2 poles (5.9547, 6.2364) (6.1326, 6.3723) (6.2586, 6.6613) (6.2586, 6.8465) knots 0 0 0 1 2 2 2
  line L169 (8.3754, 7.6937) -> (7.1823, 3.8479)
  line L170 (7.1823, 3.8479) -> (6.8365, 3.8479)
  line L171 (6.8365, 3.8479) -> (8.0246, 7.6937)
  line L172 (8.0246, 7.6937) -> (8.3754, 7.6937)
  line L173 (10.4378, 4.5099) -> (8.9509, 4.5099)
  line L174 (8.9509, 4.5099) -> (8.9509, 4.8211)
  line L175 (8.9509, 4.8211) -> (9.5042, 4.8211)
  line L176 (9.5042, 4.8211) -> (9.5042, 6.8638)
  line L177 (9.5042, 6.8638) -> (8.9509, 6.8638)
  line L178 (8.9509, 6.8638) -> (8.9509, 7.1429)
  spline S135 degree 2 poles (8.9509, 7.1429) (9.2646, 7.1429) (9.561, 7.3208) (9.5807, 7.5678) knots 0 0 0 1 2 2 2
  line L179 (9.5807, 7.5678) -> (9.8969, 7.5678)
  line L180 (9.8969, 7.5678) -> (9.8969, 4.8211)
  line L181 (9.8969, 4.8211) -> (10.4378, 4.8211)
  line L182 (10.4378, 4.8211) -> (10.4378, 4.5099)
  spline S136 degree 2 poles (11.821, 7.2689) (11.7099, 7.2689) (11.49, 7.2146) (11.3838, 7.1726) knots 0 0 0 1 2 2 2
  spline S137 degree 2 poles (11.3838, 7.1726) (11.285, 7.1306) (11.1393, 7.0417) (11.0825, 7.0021) knots 0 0 0 1 2 2 2
  line L183 (11.0825, 7.0021) -> (11.0578, 7.0021)
  line L184 (11.0578, 7.0021) -> (11.0578, 7.4344)
  spline S138 degree 2 poles (11.0578, 7.4344) (11.1912, 7.506) (11.6481, 7.6221) (11.8531, 7.6221) knots 0 0 0 1 2 2 2
  spline S139 degree 2 poles (11.8531, 7.6221) (12.0606, 7.6221) (12.3694, 7.5381) (12.4953, 7.4492) knots 0 0 0 1 2 2 2
  spline S140 degree 2 poles (12.4953, 7.4492) (12.6287, 7.3529) (12.767, 7.0738) (12.767, 6.8861) knots 0 0 0 1 2 2 2
  spline S141 degree 2 poles (12.767, 6.8861) (12.767, 6.6341) (12.4361, 6.2537) (12.2039, 6.2043) knots 0 0 0 1 2 2 2
  line L185 (12.2039, 6.2043) -> (12.2039, 6.1747)
  spline S142 degree 2 poles (12.2039, 6.1747) (12.3002, 6.1549) (12.52, 6.066) (12.6139, 5.9771) knots 0 0 0 1 2 2 2
  spline S143 degree 2 poles (12.6139, 5.9771) (12.7078, 5.8906) (12.8263, 5.614) (12.8263, 5.4139) knots 0 0 0 1 2 2 2
  spline S144 degree 2 poles (12.8263, 5.4139) (12.8263, 5.2089) (12.6855, 4.8606) (12.5571, 4.7273) knots 0 0 0 1 2 2 2
  spline S145 degree 2 poles (12.5571, 4.7273) (12.4237, 4.5889) (12.0458, 4.4457) (11.8062, 4.4457) knots 0 0 0 1 2 2 2
  spline S146 degree 2 poles (11.8062, 4.4457) (11.5765, 4.4457) (11.127, 4.5568) (10.9738, 4.6334) knots 0 0 0 1 2 2 2
  line L186 (10.9738, 4.6334) -> (10.9738, 5.0657)
  line L187 (10.9738, 5.0657) -> (11.0035, 5.0657)
  spline S147 degree 2 poles (11.0035, 5.0657) (11.1319, 4.9718) (11.5666, 4.7989) (11.7815, 4.7989) knots 0 0 0 1 2 2 2
  spline S148 degree 2 poles (11.7815, 4.7989) (11.9075, 4.7989) (12.1594, 4.8779) (12.2434, 4.9693) knots 0 0 0 1 2 2 2
  spline S149 degree 2 poles (12.2434, 4.9693) (12.3249, 5.0607) (12.4114, 5.2781) (12.4114, 5.4436) knots 0 0 0 1 2 2 2
  spline S150 degree 2 poles (12.4114, 5.4436) (12.4114, 5.6091) (12.315, 5.8239) (12.2286, 5.8857) knots 0 0 0 1 2 2 2
  spline S151 degree 2 poles (12.2286, 5.8857) (12.1421, 5.9474) (11.9075, 5.9944) (11.7692, 5.9944) knots 0 0 0 1 2 2 2
  line L188 (11.7692, 5.9944) -> (11.5963, 5.9944)
  line L189 (11.5963, 5.9944) -> (11.5963, 6.3328)
  line L190 (11.5963, 6.3328) -> (11.7321, 6.3328)
  spline S152 degree 2 poles (11.7321, 6.3328) (12.0063, 6.3328) (12.3521, 6.5946) (12.3521, 6.8441) knots 0 0 0 1 2 2 2
  spline S153 degree 2 poles (12.3521, 6.8441) (12.3521, 6.9602) (12.2632, 7.1256) (12.1915, 7.175) knots 0 0 0 1 2 2 2
  spline S154 degree 2 poles (12.1915, 7.175) (12.115, 7.2269) (11.9272, 7.2689) (11.821, 7.2689) knots 0 0 0 1 2 2 2
  line L191 (14.5529, 7.6937) -> (13.3598, 3.8479)
  line L192 (13.3598, 3.8479) -> (13.014, 3.8479)
  line L193 (13.014, 3.8479) -> (14.2021, 7.6937)
  line L194 (14.2021, 7.6937) -> (14.5529, 7.6937)
  line L195 (16.7685, 4.5099) -> (14.8888, 4.5099)
  line L196 (14.8888, 4.5099) -> (14.8888, 4.9422)
  spline S155 degree 2 poles (14.8888, 4.9422) (15.0913, 5.1323) (15.452, 5.4856) (15.6249, 5.6757) knots 0 0 0 1 2 2 2
  spline S156 degree 2 poles (15.6249, 5.6757) (15.9731, 6.0586) (16.2275, 6.518) (16.2275, 6.7626) knots 0 0 0 1 2 2 2
  spline S157 degree 2 poles (16.2275, 6.7626) (16.2275, 6.891) (16.1485, 7.0837) (16.0769, 7.1454) knots 0 0 0 1 2 2 2
  spline S158 degree 2 poles (16.0769, 7.1454) (16.0052, 7.2072) (15.8175, 7.2689) (15.7039, 7.2689) knots 0 0 0 1 2 2 2
  spline S159 degree 2 poles (15.7039, 7.2689) (15.5952, 7.2689) (15.3729, 7.2146) (15.2716, 7.1726) knots 0 0 0 1 2 2 2
  spline S160 degree 2 poles (15.2716, 7.1726) (15.1852, 7.138) (15.0246, 7.0392) (14.9752, 7.0046) knots 0 0 0 1 2 2 2
  line L197 (14.9752, 7.0046) -> (14.953, 7.0046)
  line L198 (14.953, 7.0046) -> (14.953, 7.4393)
  spline S161 degree 2 poles (14.953, 7.4393) (15.079, 7.5011) (15.531, 7.6221) (15.7335, 7.6221) knots 0 0 0 1 2 2 2
  spline S162 degree 2 poles (15.7335, 7.6221) (16.1608, 7.6221) (16.6425, 7.1701) (16.6425, 6.7848) knots 0 0 0 1 2 2 2
  spline S163 degree 2 poles (16.6425, 6.7848) (16.6425, 6.6045) (16.5585, 6.3031) (16.4844, 6.1747) knots 0 0 0 1 2 2 2
  spline S164 degree 2 poles (16.4844, 6.1747) (16.4103, 6.0413) (16.1954, 5.7795) (16.0769, 5.6535) knots 0 0 0 1 2 2 2
  spline S165 degree 2 poles (16.0769, 5.6535) (15.8842, 5.4436) (15.4124, 4.994) (15.2716, 4.8631) knots 0 0 0 1 2 2 2
  line L199 (15.2716, 4.8631) -> (16.7685, 4.8631)
  line L200 (16.7685, 4.8631) -> (16.7685, 4.5099)
  spline S166 degree 2 poles (19.0236, 5.4781) (19.0236, 5.2583) (18.8828, 4.8829) (18.7544, 4.7446) knots 0 0 0 1 2 2 2
  spline S167 degree 2 poles (18.7544, 4.7446) (18.6259, 4.6062) (18.2431, 4.4457) (18.0059, 4.4457) knots 0 0 0 1 2 2 2
  spline S168 degree 2 poles (18.0059, 4.4457) (17.7886, 4.4457) (17.3637, 4.542) (17.2081, 4.6186) knots 0 0 0 1 2 2 2
  line L201 (17.2081, 4.6186) -> (17.2081, 5.0508)
  line L202 (17.2081, 5.0508) -> (17.2378, 5.0508)
  spline S169 degree 2 poles (17.2378, 5.0508) (17.2847, 5.0163) (17.4601, 4.9273) (17.5663, 4.8878) knots 0 0 0 1 2 2 2
  spline S170 degree 2 poles (17.5663, 4.8878) (17.6873, 4.8458) (17.8874, 4.7989) (18.0134, 4.7989) knots 0 0 0 1 2 2 2
  spline S171 degree 2 poles (18.0134, 4.7989) (18.1369, 4.7989) (18.369, 4.8878) (18.453, 4.9841) knots 0 0 0 1 2 2 2
  spline S172 degree 2 poles (18.453, 4.9841) (18.5296, 5.0755) (18.6086, 5.3176) (18.6086, 5.4806) knots 0 0 0 1 2 2 2
  spline S173 degree 2 poles (18.6086, 5.4806) (18.6086, 5.6436) (18.5197, 5.8511) (18.4357, 5.9203) knots 0 0 0 1 2 2 2
  spline S174 degree 2 poles (18.4357, 5.9203) (18.3493, 5.9968) (18.0924, 6.0611) (17.9368, 6.0611) knots 0 0 0 1 2 2 2
  spline S175 degree 2 poles (17.9368, 6.0611) (17.7688, 6.0611) (17.4354, 6.0092) (17.3341, 5.987) knots 0 0 0 1 2 2 2
  line L203 (17.3341, 5.987) -> (17.3341, 7.5579)
  line L204 (17.3341, 7.5579) -> (19.0063, 7.5579)
  line L205 (19.0063, 7.5579) -> (19.0063, 7.1997)
  line L206 (19.0063, 7.1997) -> (17.7268, 7.1997)
  line L207 (17.7268, 7.1997) -> (17.7268, 6.3871)
  spline S176 degree 2 poles (17.7268, 6.3871) (17.8009, 6.397) (17.9442, 6.4044) (18.0035, 6.4044) knots 0 0 0 1 2 2 2
  spline S177 degree 2 poles (18.0035, 6.4044) (18.2381, 6.4044) (18.5617, 6.3278) (18.7099, 6.2142) knots 0 0 0 1 2 2 2
  spline S178 degree 2 poles (18.7099, 6.2142) (18.8606, 6.1006) (19.0236, 5.7548) (19.0236, 5.4781) knots 0 0 0 1 2 2 2
  point P0 (44, -10)
  dimension "d0" = 115
  dimension "d1" = 115
  constraints: 2 other
extrude "Extrusion3" cut sketch "Sketch6" against normal blind 2
equation "\"d153\" = d124"
equation "\"d124\" = 34.641016"
body "Solid1"
